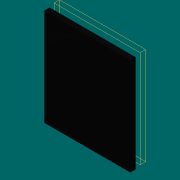
# Autodesk Inventor part: front
Saved by Autodesk Inventor 2016 (Build 200138000, 138)
## iProperties
Created: 2015-10-13
Part Number: front
Material: PC/ABS Plastic
Document SubType Name: Modeling
Designer: Sawaiz
Density: 0.357273 g/cm^3
Appearance: Smooth - Black
Author: Sawaiz
Autodesk Inventor part; units mm, degrees
ref_plane "YZ Plane" through (0, 0, 0) normal (1, 0, 0) x (0, 1, 0)
ref_plane "XZ Plane" through (0, 0, 0) normal (0, 1, 0) x (-1, 0, 0)
ref_plane "XY Plane" through (0, 0, 0) normal (0, 0, 1) x (1, 0, 0)
sketch "Sketch1" plane through (0, 0, 0) normal (1, 0, 0) x (0, 1, 0)
  line L0 (-50, -56.35) -> (50, -56.35)
  line L1 (50, -56.35) -> (50, 56.35)
  line L2 (50, 56.35) -> (-50, 56.35)
  line L3 (-50, 56.35) -> (-50, -56.35)
  line L4 (-50, -56.35) -> (50, 56.35) construction
  line L5 (50, -56.35) -> (-50, 56.35) construction
  point P0 (0, 0)
  dimension "d0" = 100
  dimension "d1" = 112.7
  constraints: 12 end point, 2 midpoint, 2 parallel, 1 horizontal, 1 perpendicular
  measures "d0" distance of L2.end L1.end
  measures "d1" distance of L1.end L0.end
extrude "Extrusion1" add sketch "Sketch1" along normal blind 6.35
equation "\"d0\" = width"
equation "\"d1\" = height + 2 * acrylicThickness"
equation "\"d2\" = acrylicThickness"
equation "\"acrylicThickness\" = 6.35"
equation "\"width\" = 100"
equation "\"mirrorAngle\" = 5deg"
equation "\"detectorWidth\" = 52"
equation "\"detectorHeight\" = 52"
equation "\"mirrorThickness\" = 3"
equation "\"fresnelThickness\" = 0.1"
equation "\"ior\" = 1.49"
equation "\"focalLength\" = 76.2"
equation "\"fresnelAngle\" = 90deg"
equation "\"centerThickness\" = 1.524"
equation "\"fresnelEffectiveDiameter\" = 76.2"
equation "\"height\" = 100"
body "Solid1"
